Autodesk Inventor part; units mm, degrees
(part 2 of 3)
  spline S276 degree 2 poles (76.7813, 10.5842) (76.5936, 10.7868) (76.3861, 11.3302) (76.3861, 11.6859) knots 0 0 0 1 2 2 2
  spline S277 degree 2 poles (76.3861, 11.6859) (76.3861, 12.4269) (77.542, 13.4297) (78.4362, 13.4297) knots 0 0 0 1 2 2 2
  spline S278 degree 2 poles (78.4362, 13.4297) (78.95, 13.4297) (79.8589, 13.2272) (80.2492, 13.0345) knots 0 0 0 1 2 2 2
  line L270 (80.2492, 13.0345) -> (80.2492, 12.0662)
  line L271 (80.2492, 12.0662) -> (80.1899, 12.0662)
  spline S279 degree 2 poles (80.1899, 12.0662) (79.8984, 12.333) (78.9895, 12.7282) (78.4905, 12.7282) knots 0 0 0 1 2 2 2
  spline S280 degree 2 poles (78.4905, 12.7282) (77.9274, 12.7282) (77.2308, 12.1996) (77.2308, 11.7698) knots 0 0 0 1 2 2 2
  spline S281 degree 2 poles (77.2308, 11.7698) (77.2308, 11.3845) (77.6408, 10.9251) (78.0262, 10.8214) knots 0 0 0 1 2 2 2
  spline S282 degree 2 poles (78.0262, 10.8214) (78.283, 10.7522) (79.029, 10.5744) (79.276, 10.5003) knots 0 0 0 1 2 2 2
  spline S283 degree 2 poles (79.276, 10.5003) (79.9034, 10.3076) (80.4863, 9.532) (80.4863, 8.9639) knots 0 0 0 1 2 2 2
  spline S284 degree 2 poles (80.4863, 8.9639) (80.4863, 8.6033) (80.1948, 7.9117) (79.933, 7.6696) knots 0 0 0 1 2 2 2
  spline S285 degree 2 poles (79.933, 7.6696) (79.6416, 7.4029) (78.9006, 7.1163) (78.3423, 7.1163) knots 0 0 0 1 2 2 2
  line L272 (87.2097, 7.225) -> (84.2358, 7.225)
  line L273 (84.2358, 7.225) -> (84.2358, 7.8475)
  line L274 (84.2358, 7.8475) -> (85.3424, 7.8475)
  line L275 (85.3424, 7.8475) -> (85.3424, 11.9329)
  line L276 (85.3424, 11.9329) -> (84.2358, 11.9329)
  line L277 (84.2358, 11.9329) -> (84.2358, 12.4911)
  spline S286 degree 2 poles (84.2358, 12.4911) (84.8632, 12.4911) (85.456, 12.8468) (85.4955, 13.3408) knots 0 0 0 1 2 2 2
  line L278 (85.4955, 13.3408) -> (86.1278, 13.3408)
  line L279 (86.1278, 13.3408) -> (86.1278, 7.8475)
  line L280 (86.1278, 7.8475) -> (87.2097, 7.8475)
  line L281 (87.2097, 7.8475) -> (87.2097, 7.225)
  line L282 (87.8469, 7.225) -> (89.902, 13.321)
  line L283 (89.902, 13.321) -> (90.8999, 13.321)
  line L284 (90.8999, 13.321) -> (92.9549, 7.225)
  line L285 (92.9549, 7.225) -> (92.1003, 7.225)
  line L286 (92.1003, 7.225) -> (91.547, 8.9293)
  line L287 (91.547, 8.9293) -> (89.2203, 8.9293)
  line L288 (89.2203, 8.9293) -> (88.667, 7.225)
  line L289 (88.667, 7.225) -> (87.8469, 7.225)
  line L290 (91.3247, 9.6209) -> (90.3812, 12.4911)
  line L291 (90.3812, 12.4911) -> (89.4426, 9.6209)
  line L292 (89.4426, 9.6209) -> (91.3247, 9.6209)
  spline S287 degree 2 poles (97.8505, 7.1163) (97.1886, 7.1163) (96.2598, 7.393) (95.8498, 7.5906) knots 0 0 0 1 2 2 2
  line L293 (95.8498, 7.5906) -> (95.8498, 8.6082)
  line L294 (95.8498, 8.6082) -> (95.9091, 8.6082)
  spline S288 degree 2 poles (95.9091, 8.6082) (96.3092, 8.2328) (97.3219, 7.8178) (97.7912, 7.8178) knots 0 0 0 1 2 2 2
  spline S289 degree 2 poles (97.7912, 7.8178) (98.4631, 7.8178) (99.1497, 8.376) (99.1497, 8.8355) knots 0 0 0 1 2 2 2
  spline S290 degree 2 poles (99.1497, 8.8355) (99.1497, 9.201) (98.7891, 9.6555) (98.3989, 9.7691) knots 0 0 0 1 2 2 2
  spline S291 degree 2 poles (98.3989, 9.7691) (98.1173, 9.8482) (97.648, 9.9569) (97.2972, 10.0458) knots 0 0 0 1 2 2 2
  spline S292 degree 2 poles (97.2972, 10.0458) (96.9811, 10.1298) (96.4821, 10.3817) (96.2895, 10.5842) knots 0 0 0 1 2 2 2
  spline S293 degree 2 poles (96.2895, 10.5842) (96.1017, 10.7868) (95.8943, 11.3302) (95.8943, 11.6859) knots 0 0 0 1 2 2 2
  spline S294 degree 2 poles (95.8943, 11.6859) (95.8943, 12.4269) (97.0502, 13.4297) (97.9444, 13.4297) knots 0 0 0 1 2 2 2
  spline S295 degree 2 poles (97.9444, 13.4297) (98.4581, 13.4297) (99.3671, 13.2272) (99.7574, 13.0345) knots 0 0 0 1 2 2 2
  line L295 (99.7574, 13.0345) -> (99.7574, 12.0662)
  line L296 (99.7574, 12.0662) -> (99.6981, 12.0662)
  spline S296 degree 2 poles (99.6981, 12.0662) (99.4066, 12.333) (98.4977, 12.7282) (97.9987, 12.7282) knots 0 0 0 1 2 2 2
  spline S297 degree 2 poles (97.9987, 12.7282) (97.4356, 12.7282) (96.739, 12.1996) (96.739, 11.7698) knots 0 0 0 1 2 2 2
  spline S298 degree 2 poles (96.739, 11.7698) (96.739, 11.3845) (97.149, 10.9251) (97.5344, 10.8214) knots 0 0 0 1 2 2 2
  spline S299 degree 2 poles (97.5344, 10.8214) (97.7912, 10.7522) (98.5372, 10.5744) (98.7842, 10.5003) knots 0 0 0 1 2 2 2
  spline S300 degree 2 poles (98.7842, 10.5003) (99.4116, 10.3076) (99.9945, 9.532) (99.9945, 8.9639) knots 0 0 0 1 2 2 2
  spline S301 degree 2 poles (99.9945, 8.9639) (99.9945, 8.6033) (99.703, 7.9117) (99.4412, 7.6696) knots 0 0 0 1 2 2 2
  spline S302 degree 2 poles (99.4412, 7.6696) (99.1497, 7.4029) (98.4087, 7.1163) (97.8505, 7.1163) knots 0 0 0 1 2 2 2
  spline S303 degree 2 poles (102.7461, 7.1213) (101.6494, 7.1213) (100.444, 8.3513) (100.444, 9.4875) knots 0 0 0 1 2 2 2
  spline S304 degree 2 poles (100.444, 9.4875) (100.444, 10.604) (101.6148, 11.9279) (102.5584, 11.9279) knots 0 0 0 1 2 2 2
  spline S305 degree 2 poles (102.5584, 11.9279) (102.9832, 11.9279) (103.6402, 11.6809) (103.8823, 11.4191) knots 0 0 0 1 2 2 2
  spline S306 degree 2 poles (103.8823, 11.4191) (104.1293, 11.1573) (104.3911, 10.4015) (104.3911, 9.8531) knots 0 0 0 1 2 2 2
  line L297 (104.3911, 9.8531) -> (104.3911, 9.4332)
  line L298 (104.3911, 9.4332) -> (101.2246, 9.4332)
  spline S307 degree 2 poles (101.2246, 9.4332) (101.2246, 8.6379) (102.0248, 7.7931) (102.7362, 7.7931) knots 0 0 0 1 2 2 2
  spline S308 degree 2 poles (102.7362, 7.7931) (102.9881, 7.7931) (103.4772, 7.9067) (103.6748, 7.9957) knots 0 0 0 1 2 2 2
  spline S309 degree 2 poles (103.6748, 7.9957) (103.8823, 8.0945) (104.1688, 8.2674) (104.2627, 8.3464) knots 0 0 0 1 2 2 2
  line L299 (104.2627, 8.3464) -> (104.3071, 8.3464)
  line L300 (104.3071, 8.3464) -> (104.3071, 7.5066)
  spline S310 degree 2 poles (104.3071, 7.5066) (104.1738, 7.4523) (103.7687, 7.2942) (103.6106, 7.2497) knots 0 0 0 1 2 2 2
  spline S311 degree 2 poles (103.6106, 7.2497) (103.3883, 7.1855) (103.0227, 7.1213) (102.7461, 7.1213) knots 0 0 0 1 2 2 2
  spline S312 degree 2 poles (103.6402, 10.0211) (103.6304, 10.3323) (103.5019, 10.7868) (103.3784, 10.9399) knots 0 0 0 1 2 2 2
  spline S313 degree 2 poles (103.3784, 10.9399) (103.245, 11.1128) (102.8251, 11.2956) (102.5139, 11.2956) knots 0 0 0 1 2 2 2
  spline S314 degree 2 poles (102.5139, 11.2956) (102.2076, 11.2956) (101.7778, 11.1128) (101.6, 10.935) knots 0 0 0 1 2 2 2
  spline S315 degree 2 poles (101.6, 10.935) (101.4271, 10.7522) (101.2493, 10.3125) (101.2246, 10.0211) knots 0 0 0 1 2 2 2
  line L301 (101.2246, 10.0211) -> (103.6402, 10.0211)
  spline S316 degree 2 poles (106.9896, 7.1213) (106.5153, 7.1213) (105.7299, 7.4127) (105.4483, 7.7091) knots 0 0 0 1 2 2 2
  spline S317 degree 2 poles (105.4483, 7.7091) (105.1667, 8.0006) (104.8555, 8.8997) (104.8555, 9.5024) knots 0 0 0 1 2 2 2
  spline S318 degree 2 poles (104.8555, 9.5024) (104.8555, 10.1051) (105.1766, 10.9844) (105.4483, 11.2808) knots 0 0 0 1 2 2 2
  spline S319 degree 2 poles (105.4483, 11.2808) (105.72, 11.5821) (106.5252, 11.9032) (106.9896, 11.9032) knots 0 0 0 1 2 2 2
  spline S320 degree 2 poles (106.9896, 11.9032) (107.365, 11.9032) (108.0665, 11.6908) (108.3382, 11.5525) knots 0 0 0 1 2 2 2
  line L302 (108.3382, 11.5525) -> (108.3382, 10.688)
  line L303 (108.3382, 10.688) -> (108.2937, 10.688)
  spline S321 degree 2 poles (108.2937, 10.688) (108.2098, 10.7571) (107.9529, 10.935) (107.7701, 11.0288) knots 0 0 0 1 2 2 2
  spline S322 degree 2 poles (107.7701, 11.0288) (107.6071, 11.1079) (107.1724, 11.2314) (106.9748, 11.2314) knots 0 0 0 1 2 2 2
  spline S323 degree 2 poles (106.9748, 11.2314) (106.377, 11.2314) (105.6508, 10.3274) (105.6508, 9.5024) knots 0 0 0 1 2 2 2
  spline S324 degree 2 poles (105.6508, 9.5024) (105.6508, 8.6971) (106.3523, 7.7931) (106.9748, 7.7931) knots 0 0 0 1 2 2 2
  spline S325 degree 2 poles (106.9748, 7.7931) (107.3502, 7.7931) (108.0319, 8.1043) (108.2937, 8.3464) knots 0 0 0 1 2 2 2
  line L304 (108.2937, 8.3464) -> (108.3382, 8.3464)
  line L305 (108.3382, 8.3464) -> (108.3382, 7.4819)
  spline S326 degree 2 poles (108.3382, 7.4819) (108.2246, 7.4276) (107.8788, 7.2744) (107.7405, 7.2398) knots 0 0 0 1 2 2 2
  spline S327 degree 2 poles (107.7405, 7.2398) (107.5429, 7.1806) (107.2316, 7.1213) (106.9896, 7.1213) knots 0 0 0 1 2 2 2
  spline S328 degree 2 poles (110.4229, 7.1361) (109.7955, 7.1361) (109.0891, 7.8524) (109.0891, 8.628) knots 0 0 0 1 2 2 2
  line L306 (109.0891, 8.628) -> (109.0891, 11.1622)
  line L307 (109.0891, 11.1622) -> (108.5704, 11.1622)
  line L308 (108.5704, 11.1622) -> (108.5704, 11.7995)
  line L309 (108.5704, 11.7995) -> (109.0891, 11.7995)
  line L310 (109.0891, 11.7995) -> (109.0891, 13.1135)
  line L311 (109.0891, 13.1135) -> (109.8597, 13.1135)
  line L312 (109.8597, 13.1135) -> (109.8597, 11.7995)
  line L313 (109.8597, 11.7995) -> (111.2775, 11.7995)
  line L314 (111.2775, 11.7995) -> (111.2775, 11.1622)
  line L315 (111.2775, 11.1622) -> (109.8597, 11.1622)
  line L316 (109.8597, 11.1622) -> (109.8597, 8.9837)
  spline S329 degree 2 poles (109.8597, 8.9837) (109.8597, 8.6379) (109.8844, 8.2575) (109.9684, 8.0945) knots 0 0 0 1 2 2 2
  spline S330 degree 2 poles (109.9684, 8.0945) (110.0376, 7.9512) (110.3488, 7.8079) (110.6156, 7.8079) knots 0 0 0 1 2 2 2
  spline S331 degree 2 poles (110.6156, 7.8079) (110.8033, 7.8079) (111.154, 7.9216) (111.2331, 7.9561) knots 0 0 0 1 2 2 2
  line L317 (111.2331, 7.9561) -> (111.2775, 7.9561)
  line L318 (111.2775, 7.9561) -> (111.2775, 7.2645)
  spline S332 degree 2 poles (111.2775, 7.2645) (111.0602, 7.2053) (110.6156, 7.1361) (110.4229, 7.1361) knots 0 0 0 1 2 2 2
  line L319 (112.6311, 7.225) -> (111.8604, 7.225)
  line L320 (111.8604, 7.225) -> (111.8604, 11.7995)
  line L321 (111.8604, 11.7995) -> (112.6311, 11.7995)
  line L322 (112.6311, 11.7995) -> (112.6311, 7.225)
  line L323 (112.6854, 12.5602) -> (111.811, 12.5602)
  line L324 (111.811, 12.5602) -> (111.811, 13.3605)
  line L325 (111.811, 13.3605) -> (112.6854, 13.3605)
  line L326 (112.6854, 13.3605) -> (112.6854, 12.5602)
  spline S333 degree 2 poles (117.5217, 9.5122) (117.5217, 8.3563) (116.4102, 7.0966) (115.4815, 7.0966) knots 0 0 0 1 2 2 2
  spline S334 degree 2 poles (115.4815, 7.0966) (114.5281, 7.0966) (113.4363, 8.3958) (113.4363, 9.5122) knots 0 0 0 1 2 2 2
  spline S335 degree 2 poles (113.4363, 9.5122) (113.4363, 10.6583) (114.5626, 11.9279) (115.4815, 11.9279) knots 0 0 0 1 2 2 2
  spline S336 degree 2 poles (115.4815, 11.9279) (116.4102, 11.9279) (117.5217, 10.6633) (117.5217, 9.5122) knots 0 0 0 1 2 2 2
  spline S337 degree 2 poles (116.7264, 9.5122) (116.7264, 10.4015) (116.0792, 11.266) (115.4815, 11.266) knots 0 0 0 1 2 2 2
  spline S338 degree 2 poles (115.4815, 11.266) (114.8837, 11.266) (114.2317, 10.4015) (114.2317, 9.5122) knots 0 0 0 1 2 2 2
  spline S339 degree 2 poles (114.2317, 9.5122) (114.2317, 8.6477) (114.8837, 7.7585) (115.4815, 7.7585) knots 0 0 0 1 2 2 2
  spline S340 degree 2 poles (115.4815, 7.7585) (116.0743, 7.7585) (116.7264, 8.6329) (116.7264, 9.5122) knots 0 0 0 1 2 2 2
  line L327 (121.9035, 7.225) -> (121.1329, 7.225)
  line L328 (121.1329, 7.225) -> (121.1329, 9.8334)
  spline S341 degree 2 poles (121.1329, 9.8334) (121.1329, 10.1495) (121.0736, 10.6929) (120.9847, 10.8559) knots 0 0 0 1 2 2 2
  spline S342 degree 2 poles (120.9847, 10.8559) (120.8908, 11.0288) (120.5549, 11.1968) (120.2684, 11.1968) knots 0 0 0 1 2 2 2
  spline S343 degree 2 poles (120.2684, 11.1968) (119.9819, 11.1968) (119.3742, 10.8905) (119.0828, 10.6435) knots 0 0 0 1 2 2 2
  line L329 (119.0828, 10.6435) -> (119.0828, 7.225)
  line L330 (119.0828, 7.225) -> (118.3121, 7.225)
  line L331 (118.3121, 7.225) -> (118.3121, 11.7995)
  line L332 (118.3121, 11.7995) -> (119.0828, 11.7995)
  line L333 (119.0828, 11.7995) -> (119.0828, 11.2907)
  spline S344 degree 2 poles (119.0828, 11.2907) (119.4286, 11.6019) (120.0955, 11.9279) (120.4709, 11.9279) knots 0 0 0 1 2 2 2
  spline S345 degree 2 poles (120.4709, 11.9279) (121.1428, 11.9279) (121.9035, 11.0387) (121.9035, 10.194) knots 0 0 0 1 2 2 2
  line L334 (121.9035, 10.194) -> (121.9035, 7.225)
  spline S346 degree 2 poles (129.7977, 9.0973) (129.7977, 8.6428) (129.4519, 7.9463) (129.1654, 7.719) knots 0 0 0 1 2 2 2
  spline S347 degree 2 poles (129.1654, 7.719) (128.8196, 7.4523) (128.0341, 7.225) (127.4117, 7.225) knots 0 0 0 1 2 2 2
  line L335 (127.4117, 7.225) -> (125.6629, 7.225)
  line L336 (125.6629, 7.225) -> (125.6629, 13.321)
  line L337 (125.6629, 13.321) -> (127.2783, 13.321)
  spline S348 degree 2 poles (127.2783, 13.321) (127.9304, 13.321) (128.5825, 13.237) (128.8789, 13.074) knots 0 0 0 1 2 2 2
  spline S349 degree 2 poles (128.8789, 13.074) (129.2098, 12.9011) (129.5112, 12.333) (129.5112, 11.9477) knots 0 0 0 1 2 2 2
  spline S350 degree 2 poles (129.5112, 11.9477) (129.5112, 11.5179) (129.0567, 10.8362) (128.6566, 10.6435) knots 0 0 0 1 2 2 2
  line L338 (128.6566, 10.6435) -> (128.6566, 10.6139)
  spline S351 degree 2 poles (128.6566, 10.6139) (129.2, 10.4657) (129.7977, 9.6802) (129.7977, 9.0973) knots 0 0 0 1 2 2 2
  spline S352 degree 2 poles (128.953, 9.0627) (128.953, 9.4085) (128.7554, 9.8531) (128.459, 10.0112) knots 0 0 0 1 2 2 2
  spline S353 degree 2 poles (128.459, 10.0112) (128.2663, 10.11) (127.8118, 10.1693) (127.3919, 10.1693) knots 0 0 0 1 2 2 2
  line L339 (127.3919, 10.1693) -> (126.4731, 10.1693)
  line L340 (126.4731, 10.1693) -> (126.4731, 7.9166)
  line L341 (126.4731, 7.9166) -> (127.1301, 7.9166)
  spline S354 degree 2 poles (127.1301, 7.9166) (127.6636, 7.9166) (128.2762, 8.0154) (128.5133, 8.1735) knots 0 0 0 1 2 2 2
  spline S355 degree 2 poles (128.5133, 8.1735) (128.7405, 8.3365) (128.953, 8.7416) (128.953, 9.0627) knots 0 0 0 1 2 2 2
  spline S356 degree 2 poles (128.6664, 11.8341) (128.6664, 12.0514) (128.5182, 12.3775) (128.3552, 12.4713) knots 0 0 0 1 2 2 2
  spline S357 degree 2 poles (128.3552, 12.4713) (128.1576, 12.58) (127.6784, 12.6294) (127.2486, 12.6294) knots 0 0 0 1 2 2 2
  line L342 (127.2486, 12.6294) -> (126.4731, 12.6294)
  line L343 (126.4731, 12.6294) -> (126.4731, 10.8461)
  line L344 (126.4731, 10.8461) -> (127.3919, 10.8461)
  spline S358 degree 2 poles (127.3919, 10.8461) (127.7723, 10.8461) (128.1329, 10.9251) (128.3256, 11.0486) knots 0 0 0 1 2 2 2
  spline S359 degree 2 poles (128.3256, 11.0486) (128.5133, 11.1672) (128.6664, 11.5475) (128.6664, 11.8341) knots 0 0 0 1 2 2 2
  spline S360 degree 2 poles (134.224, 10.273) (134.224, 8.6329) (133.2705, 7.0966) (132.2776, 7.0966) knots 0 0 0 1 2 2 2
  spline S361 degree 2 poles (132.2776, 7.0966) (131.2698, 7.0966) (130.3263, 8.6626) (130.3263, 10.2681) knots 0 0 0 1 2 2 2
  spline S362 degree 2 poles (130.3263, 10.2681) (130.3263, 11.918) (131.2797, 13.4445) (132.2776, 13.4445) knots 0 0 0 1 2 2 2
  spline S363 degree 2 poles (132.2776, 13.4445) (133.2804, 13.4445) (134.224, 11.8637) (134.224, 10.273) knots 0 0 0 1 2 2 2
  spline S364 degree 2 poles (133.1767, 8.4156) (133.2952, 8.7169) (133.394, 9.6456) (133.394, 10.273) knots 0 0 0 1 2 2 2
  spline S365 degree 2 poles (133.394, 10.273) (133.394, 10.9004) (133.2952, 11.8242) (133.1717, 12.1354) knots 0 0 0 1 2 2 2
  spline S366 degree 2 poles (133.1717, 12.1354) (133.0482, 12.4466) (132.6185, 12.7677) (132.2776, 12.7677) knots 0 0 0 1 2 2 2
  spline S367 degree 2 poles (132.2776, 12.7677) (131.9367, 12.7677) (131.4971, 12.4466) (131.3686, 12.1255) knots 0 0 0 1 2 2 2
  spline S368 degree 2 poles (131.3686, 12.1255) (131.2451, 11.8143) (131.1562, 10.8658) (131.1562, 10.2681) knots 0 0 0 1 2 2 2
  spline S369 degree 2 poles (131.1562, 10.2681) (131.1562, 9.6259) (131.2353, 8.7663) (131.3637, 8.4304) knots 0 0 0 1 2 2 2
  spline S370 degree 2 poles (131.3637, 8.4304) (131.4823, 8.1142) (131.9219, 7.7734) (132.2776, 7.7734) knots 0 0 0 1 2 2 2
  spline S371 degree 2 poles (132.2776, 7.7734) (132.6135, 7.7734) (133.0532, 8.0945) (133.1767, 8.4156) knots 0 0 0 1 2 2 2
  spline S372 degree 2 poles (136.6495, 12.743) (136.4272, 12.743) (135.9876, 12.6343) (135.7751, 12.5504) knots 0 0 0 1 2 2 2
  spline S373 degree 2 poles (135.7751, 12.5504) (135.5775, 12.4664) (135.2861, 12.2885) (135.1725, 12.2095) knots 0 0 0 1 2 2 2
  line L345 (135.1725, 12.2095) -> (135.1231, 12.2095)
  line L346 (135.1231, 12.2095) -> (135.1231, 13.074)
  spline S374 degree 2 poles (135.1231, 13.074) (135.3898, 13.2173) (136.3037, 13.4495) (136.7138, 13.4495) knots 0 0 0 1 2 2 2
  spline S375 degree 2 poles (136.7138, 13.4495) (137.1287, 13.4495) (137.7462, 13.2815) (137.9982, 13.1037) knots 0 0 0 1 2 2 2
  spline S376 degree 2 poles (137.9982, 13.1037) (138.2649, 12.911) (138.5416, 12.3528) (138.5416, 11.9773) knots 0 0 0 1 2 2 2
  spline S377 degree 2 poles (138.5416, 11.9773) (138.5416, 11.4734) (137.8796, 10.7127) (137.4152, 10.6139) knots 0 0 0 1 2 2 2
  line L347 (137.4152, 10.6139) -> (137.4152, 10.5546)
  spline S378 degree 2 poles (137.4152, 10.5546) (137.6079, 10.5151) (138.0476, 10.3372) (138.2353, 10.1594) knots 0 0 0 1 2 2 2
  spline S379 degree 2 poles (138.2353, 10.1594) (138.423, 9.9865) (138.6601, 9.4332) (138.6601, 9.0331) knots 0 0 0 1 2 2 2
  spline S380 degree 2 poles (138.6601, 9.0331) (138.6601, 8.623) (138.3785, 7.9265) (138.1217, 7.6597) knots 0 0 0 1 2 2 2
  spline S381 degree 2 poles (138.1217, 7.6597) (137.8549, 7.3831) (137.0991, 7.0966) (136.6199, 7.0966) knots 0 0 0 1 2 2 2
  spline S382 degree 2 poles (136.6199, 7.0966) (136.1605, 7.0966) (135.2614, 7.3189) (134.9551, 7.472) knots 0 0 0 1 2 2 2
  line L348 (134.9551, 7.472) -> (134.9551, 8.3365)
  line L349 (134.9551, 8.3365) -> (135.0144, 8.3365)
  spline S383 degree 2 poles (135.0144, 8.3365) (135.2713, 8.1488) (136.1407, 7.803) (136.5705, 7.803) knots 0 0 0 1 2 2 2
  spline S384 degree 2 poles (136.5705, 7.803) (136.8224, 7.803) (137.3263, 7.9611) (137.4943, 8.1439) knots 0 0 0 1 2 2 2
  spline S385 degree 2 poles (137.4943, 8.1439) (137.6573, 8.3266) (137.8302, 8.7614) (137.8302, 9.0923) knots 0 0 0 1 2 2 2
  spline S386 degree 2 poles (137.8302, 9.0923) (137.8302, 9.4233) (137.6375, 9.8531) (137.4646, 9.9766) knots 0 0 0 1 2 2 2
  spline S387 degree 2 poles (137.4646, 9.9766) (137.2917, 10.1001) (136.8224, 10.194) (136.5458, 10.194) knots 0 0 0 1 2 2 2
  line L350 (136.5458, 10.194) -> (136.2, 10.194)
  line L351 (136.2, 10.194) -> (136.2, 10.8708)
  line L352 (136.2, 10.8708) -> (136.4717, 10.8708)
  spline S388 degree 2 poles (136.4717, 10.8708) (137.02, 10.8708) (137.7116, 11.3944) (137.7116, 11.8933) knots 0 0 0 1 2 2 2
  spline S389 degree 2 poles (137.7116, 11.8933) (137.7116, 12.1255) (137.5338, 12.4565) (137.3905, 12.5553) knots 0 0 0 1 2 2 2
  spline S390 degree 2 poles (137.3905, 12.5553) (137.2374, 12.659) (136.862, 12.743) (136.6495, 12.743) knots 0 0 0 1 2 2 2
  dimension "d2" = 50.8
  dimension "d3" = 203.2
  dimension "d4" = 50.8
  dimension "d5" = 101.6
  dimension "d6" = 8.128
  dimension "d7" = 21.336
  constraints: 2 other
  measures "d2" distance between parallel lines of L2 L7
  measures "d3" distance of L2.end L0.start
  measures "d4" distance of L1.end L2.end
  measures "d5" distance of L5.end L6.end
  measures "d6" distance of L6.end L4.start
  measures "d7" distance between parallel lines of L1 L4
extrude "Extrusion2" cut sketch "Sketch2" against normal blind 5.08 contours S0 S1 L8 L9 S2 S3 S4 L10 L11 L12 L13 L14 | L15 L16 S5 S6 S7 L17 L18 L19 S8 S9 S10 L20 L21 L22 | S11 L23 L24 S12 S13 S14 S15 S16 S17 S18 S19 S20 L25 L26 S21 S22 S23 S24 S25 S26 S27 | S28 L27 L28 L29 L30 L31 L32 L33 L34 L35 L36 L37 S29 S30 S31 L38 L39 S32 | L40 L41 L42 L43 | L44 L45 L46 L47 | L48 L49 S33 S34 S35 L50 L51 L52 L53 L54 S36 S37 L55 | L56 L57 L58 L59 L60 L61 L62 L63 | L67 L68 L69 L70 | L71 L72 L73 L74 | S38 S39 S40 S41 L75 L76 S42 S43 S44 L77 L78 S45 S46 | L80 L81 S51 S52 S53 L82 L83 L84 L85 L86 S54 S55 L87 | L88 L89 L90 L91 L92 L93 L94 L95 | L99 L100 L101 L102 L103 L104 S56 L105 L106 L107 L108 | L109 L110 L111 L112 L113 L114 L115 L116 L117 L118 L119 | S57 S58 S59 L123 L124 S60 S61 S62 S63 S64 S65 S66 L125 L126 L127 L128 L129 S67 S68 S69 | S70 S71 S72 S73 S74 S75 S76 L130 L131 S77 S78 S79 S80 S81 | S89 S90 S91 S92 S93 S94 S95 L132 L133 S96 S97 S98 S99 S100 | S108 S109 S110 S111 | L134 L135 L136 L137 L138 L139 L140 | L141 L142 L143 L144 L145 L146 S120 L147 L148 L149 L150 | S121 S122 L151 L152 S123 S124 S125 L153 L154 L155 L156 L157 | L158 L159 L160 L161 | S126 S127 L162 L163 L164 L165 L166 S128 S129 | S134 S135 S136 S137 S138 S139 L168 S140 S141 S142 L169 L170 S143 S144 S145 L171 L172 L173 | L175 L176 L177 L178 | L179 L180 L181 L182 | S150 S151 S152 S153 L183 L184 S154 S155 S156 L185 L186 S157 S158 | L188 L189 S163 S164 S165 L190 L191 L192 L193 L194 S166 S167 L195 | S168 L196 L197 S169 S170 S171 S172 L198 L199 L200 L201 S173 S174 S175 S176 S177 L202 S178 S179 S180 S181 | L204 L205 S186 S187 S188 L206 L207 L208 S189 S190 S191 L209 L210 L211 | S192 S193 S194 S195 S196 L212 L213 S197 S198 S199 S200 S201 L214 L215 S202 S203 | S204 L216 L217 S205 S206 S207 S208 S209 S210 S211 S212 S213 L218 L219 S214 S215 S216 S217 S218 S219 S220 | L220 L221 S221 S222 S223 S224 S225 S226 S227 L222 L223 L224 | L226 L227 L228 L229 | S232 S233 S234 S235 L230 L231 S236 S237 S238 L232 L233 S239 S240 | L235 L236 S245 S246 S247 S248 S249 S250 S251 L237 L238 L239 | L241 L242 S256 S257 S258 L243 L244 L245 S259 S260 S261 L246 L247 L248 | L249 L250 L251 L252 L253 L254 L255 L256 L257 L258 L259 L260 L261 | S262 S263 L262 L263 L264 S264 S265 S266 S267 L265 L266 L267 S268 S269 | S270 L268 L269 S271 S272 S273 S274 S275 S276 S277 S278 L270 L271 S279 S280 S281 S282 S283 S284 S285 | L272 L273 L274 L275 L276 L277 S286 L278 L279 L280 L281 | L282 L283 L284 L285 L286 L287 L288 L289 | S287 L293 L294 S288 S289 S290 S291 S292 S293 S294 S295 L295 L296 S296 S297 S298 S299 S300 S301 S302 | S303 S304 S305 S306 L297 L298 S307 S308 S309 L299 L300 S310 S311 | S316 S317 S318 S319 S320 L302 L303 S321 S322 S323 S324 S325 L304 L305 S326 S327 | S328 L306 L307 L308 L309 L310 L311 L312 L313 L314 L315 L316 S329 S330 S331 L317 L318 S332 | L319 L320 L321 L322 | L323 L324 L325 L326 | S333 S334 S335 S336 | L327 L328 S341 S342 S343 L329 L330 L331 L332 L333 S344 S345 L334 | S346 S347 L335 L336 L337 S348 S349 S350 L338 S351 | S360 S361 S362 S363 | S372 S373 L345 L346 S374 S375 S376 S377 L347 S378 S379 S380 S381 S382 L348 L349 S383 S384 S385 S386 S387 L350 L351 L352 S388 S389 S390
sketch "Sketch3" plane through (0, 0, 50.8) normal (0, 0, 1) x (1, 0, 0)
  line L0 (0, 0) -> (203.2, 0) projected
  line L1 (0, 0) -> (0, -25.4) projected
  line L2 (203.2, -25.4) -> (0, -25.4) projected
  line L3 (203.2, 0) -> (203.2, -25.4) projected
  line L4 (50.8, -8.636) -> (152.4, -8.636) construction
  line L5 (152.4, -8.636) -> (152.4, -16.764) construction
  line L6 (152.4, -16.764) -> (50.8, -16.764) construction
  line L7 (50.8, -16.764) -> (50.8, -8.636) construction
  line L8 (77.3469, -15.748) -> (73.8148, -15.748)
  line L9 (73.8148, -15.748) -> (73.8148, -9.652)
  line L10 (73.8148, -9.652) -> (74.625, -9.652)
  line L11 (74.625, -9.652) -> (74.625, -15.0268)
  line L12 (74.625, -15.0268) -> (77.3469, -15.0268)
  line L13 (77.3469, -15.0268) -> (77.3469, -15.748)
  line L14 (80.1084, -15.748) -> (77.7471, -15.748)
  line L15 (77.7471, -15.748) -> (77.7471, -15.1256)
  line L16 (77.7471, -15.1256) -> (78.5226, -15.1256)
  line L17 (78.5226, -15.1256) -> (78.5226, -10.2744)
  line L18 (78.5226, -10.2744) -> (77.7471, -10.2744)
  line L19 (77.7471, -10.2744) -> (77.7471, -9.652)
  line L20 (77.7471, -9.652) -> (80.1084, -9.652)
  line L21 (80.1084, -9.652) -> (80.1084, -10.2744)
  line L22 (80.1084, -10.2744) -> (79.3328, -10.2744)
  line L23 (79.3328, -10.2744) -> (79.3328, -15.1256)
  line L24 (79.3328, -15.1256) -> (80.1084, -15.1256)
  line L25 (80.1084, -15.1256) -> (80.1084, -15.748)
  spline S0 degree 2 poles (85.246, -13.8757) (85.246, -14.3302) (84.9002, -15.0268) (84.6137, -15.254) knots 0 0 0 1 2 2 2
  spline S1 degree 2 poles (84.6137, -15.254) (84.2679, -15.5208) (83.4824, -15.748) (82.86, -15.748) knots 0 0 0 1 2 2 2
  line L26 (82.86, -15.748) -> (81.1112, -15.748)
  line L27 (81.1112, -15.748) -> (81.1112, -9.652)
  line L28 (81.1112, -9.652) -> (82.7266, -9.652)
  spline S2 degree 2 poles (82.7266, -9.652) (83.3787, -9.652) (84.0308, -9.736) (84.3272, -9.899) knots 0 0 0 1 2 2 2
  spline S3 degree 2 poles (84.3272, -9.899) (84.6582, -10.0719) (84.9595, -10.64) (84.9595, -11.0253) knots 0 0 0 1 2 2 2
  spline S4 degree 2 poles (84.9595, -11.0253) (84.9595, -11.4551) (84.505, -12.1368) (84.1049, -12.3295) knots 0 0 0 1 2 2 2
  line L29 (84.1049, -12.3295) -> (84.1049, -12.3591)
  spline S5 degree 2 poles (84.1049, -12.3591) (84.6483, -12.5073) (85.246, -13.2928) (85.246, -13.8757) knots 0 0 0 1 2 2 2
  spline S6 degree 2 poles (84.4013, -13.9103) (84.4013, -13.5645) (84.2037, -13.1199) (83.9073, -12.9618) knots 0 0 0 1 2 2 2
  spline S7 degree 2 poles (83.9073, -12.9618) (83.7146, -12.863) (83.2601, -12.8037) (82.8402, -12.8037) knots 0 0 0 1 2 2 2
  line L30 (82.8402, -12.8037) -> (81.9214, -12.8037)
  line L31 (81.9214, -12.8037) -> (81.9214, -15.0564)
  line L32 (81.9214, -15.0564) -> (82.5784, -15.0564)
  spline S8 degree 2 poles (82.5784, -15.0564) (83.1119, -15.0564) (83.7245, -14.9576) (83.9616, -14.7995) knots 0 0 0 1 2 2 2
  spline S9 degree 2 poles (83.9616, -14.7995) (84.1889, -14.6365) (84.4013, -14.2314) (84.4013, -13.9103) knots 0 0 0 1 2 2 2
  spline S10 degree 2 poles (84.1148, -11.1389) (84.1148, -10.9216) (83.9666, -10.5955) (83.8035, -10.5017) knots 0 0 0 1 2 2 2
  spline S11 degree 2 poles (83.8035, -10.5017) (83.6059, -10.393) (83.1267, -10.3436) (82.697, -10.3436) knots 0 0 0 1 2 2 2
  line L33 (82.697, -10.3436) -> (81.9214, -10.3436)
  line L34 (81.9214, -10.3436) -> (81.9214, -12.127)
  line L35 (81.9214, -12.127) -> (82.8402, -12.127)
  spline S12 degree 2 poles (82.8402, -12.127) (83.2206, -12.127) (83.5812, -12.0479) (83.7739, -11.9244) knots 0 0 0 1 2 2 2
  spline S13 degree 2 poles (83.7739, -11.9244) (83.9616, -11.8059) (84.1148, -11.4255) (84.1148, -11.1389) knots 0 0 0 1 2 2 2
  line L36 (90.769, -15.748) -> (89.7167, -15.748)
  line L37 (89.7167, -15.748) -> (87.7901, -13.3224)
  line L38 (87.7901, -13.3224) -> (86.8614, -13.3224)
  line L39 (86.8614, -13.3224) -> (86.8614, -15.748)
  line L40 (86.8614, -15.748) -> (86.0512, -15.748)
  line L41 (86.0512, -15.748) -> (86.0512, -9.652)
  line L42 (86.0512, -9.652) -> (87.6222, -9.652)
  spline S14 degree 2 poles (87.6222, -9.652) (88.1458, -9.652) (88.8522, -9.7656) (89.1733, -9.9731) knots 0 0 0 1 2 2 2
  spline S15 degree 2 poles (89.1733, -9.9731) (89.4944, -10.1806) (89.865, -10.8277) (89.865, -11.3069) knots 0 0 0 1 2 2 2
  spline S16 degree 2 poles (89.865, -11.3069) (89.865, -11.9738) (89.1832, -12.8778) (88.6003, -13.0952) knots 0 0 0 1 2 2 2
  line L43 (88.6003, -13.0952) -> (90.769, -15.748)
  spline S17 degree 2 poles (89.0202, -11.3711) (89.0202, -11.1044) (88.8325, -10.6943) (88.6349, -10.561) knots 0 0 0 1 2 2 2
  spline S18 degree 2 poles (88.6349, -10.561) (88.462, -10.4473) (88.0026, -10.3535) (87.6666, -10.3535) knots 0 0 0 1 2 2 2
  line L44 (87.6666, -10.3535) -> (86.8614, -10.3535)
  line L45 (86.8614, -10.3535) -> (86.8614, -12.6457)
  line L46 (86.8614, -12.6457) -> (87.5728, -12.6457)
  spline S19 degree 2 poles (87.5728, -12.6457) (87.9235, -12.6457) (88.4817, -12.5222) (88.6744, -12.3295) knots 0 0 0 1 2 2 2
  spline S20 degree 2 poles (88.6744, -12.3295) (88.8522, -12.1615) (89.0202, -11.6873) (89.0202, -11.3711) knots 0 0 0 1 2 2 2
  line L47 (90.5961, -15.748) -> (92.6511, -9.652)
  line L48 (92.6511, -9.652) -> (93.649, -9.652)
  line L49 (93.649, -9.652) -> (95.7041, -15.748)
  line L50 (95.7041, -15.748) -> (94.8494, -15.748)
  line L51 (94.8494, -15.748) -> (94.2962, -14.0437)
  line L52 (94.2962, -14.0437) -> (91.9694, -14.0437)
  line L53 (91.9694, -14.0437) -> (91.4161, -15.748)
  line L54 (91.4161, -15.748) -> (90.5961, -15.748)
  line L55 (94.0739, -13.3521) -> (93.1303, -10.4819)
  line L56 (93.1303, -10.4819) -> (92.1917, -13.3521)
  line L57 (92.1917, -13.3521) -> (94.0739, -13.3521)
  line L58 (100.9998, -15.748) -> (99.9476, -15.748)
  line L59 (99.9476, -15.748) -> (98.0209, -13.3224)
  line L60 (98.0209, -13.3224) -> (97.0922, -13.3224)
  line L61 (97.0922, -13.3224) -> (97.0922, -15.748)
  line L62 (97.0922, -15.748) -> (96.2821, -15.748)
  line L63 (96.2821, -15.748) -> (96.2821, -9.652)
  line L64 (96.2821, -9.652) -> (97.853, -9.652)
  spline S21 degree 2 poles (97.853, -9.652) (98.3766, -9.652) (99.0831, -9.7656) (99.4042, -9.9731) knots 0 0 0 1 2 2 2
  spline S22 degree 2 poles (99.4042, -9.9731) (99.7253, -10.1806) (100.0958, -10.8277) (100.0958, -11.3069) knots 0 0 0 1 2 2 2
  spline S23 degree 2 poles (100.0958, -11.3069) (100.0958, -11.9738) (99.414, -12.8778) (98.8311, -13.0952) knots 0 0 0 1 2 2 2
  line L65 (98.8311, -13.0952) -> (100.9998, -15.748)
  spline S24 degree 2 poles (99.251, -11.3711) (99.251, -11.1044) (99.0633, -10.6943) (98.8657, -10.561) knots 0 0 0 1 2 2 2
  spline S25 degree 2 poles (98.8657, -10.561) (98.6928, -10.4473) (98.2334, -10.3535) (97.8974, -10.3535) knots 0 0 0 1 2 2 2
  line L66 (97.8974, -10.3535) -> (97.0922, -10.3535)
  line L67 (97.0922, -10.3535) -> (97.0922, -12.6457)
  line L68 (97.0922, -12.6457) -> (97.8036, -12.6457)
  spline S26 degree 2 poles (97.8036, -12.6457) (98.1543, -12.6457) (98.7125, -12.5222) (98.9052, -12.3295) knots 0 0 0 1 2 2 2
  spline S27 degree 2 poles (98.9052, -12.3295) (99.0831, -12.1615) (99.251, -11.6873) (99.251, -11.3711) knots 0 0 0 1 2 2 2
  line L69 (105.7521, -9.652) -> (103.6921, -13.0507)
  line L70 (103.6921, -13.0507) -> (103.6921, -15.748)
  line L71 (103.6921, -15.748) -> (102.8819, -15.748)
  line L72 (102.8819, -15.748) -> (102.8819, -13.1347)
  line L73 (102.8819, -13.1347) -> (100.8219, -9.652)
  line L74 (100.8219, -9.652) -> (101.721, -9.652)
  line L75 (101.721, -9.652) -> (103.292, -12.3344)
  line L76 (103.292, -12.3344) -> (104.8925, -9.652)
  line L77 (104.8925, -9.652) -> (105.7521, -9.652)
  line L78 (115.7655, -9.652) -> (114.2341, -15.748)
  line L79 (114.2341, -15.748) -> (113.3252, -15.748)
  line L80 (113.3252, -15.748) -> (112.0852, -10.6894)
  line L81 (112.0852, -10.6894) -> (110.8798, -15.748)
  line L82 (110.8798, -15.748) -> (109.9808, -15.748)
  line L83 (109.9808, -15.748) -> (108.4247, -9.652)
  line L84 (108.4247, -9.652) -> (109.2595, -9.652)
  line L85 (109.2595, -9.652) -> (110.4846, -14.7057)
  line L86 (110.4846, -14.7057) -> (111.6999, -9.652)
  line L87 (111.6999, -9.652) -> (112.5249, -9.652)
  line L88 (112.5249, -9.652) -> (113.75, -14.7649)
  line L89 (113.75, -14.7649) -> (114.9702, -9.652)
  line L90 (114.9702, -9.652) -> (115.7655, -9.652)
  line L91 (115.8347, -15.748) -> (117.8898, -9.652)
  line L92 (117.8898, -9.652) -> (118.8876, -9.652)
  line L93 (118.8876, -9.652) -> (120.9427, -15.748)
  line L94 (120.9427, -15.748) -> (120.0881, -15.748)
  line L95 (120.0881, -15.748) -> (119.5348, -14.0437)
  line L96 (119.5348, -14.0437) -> (117.208, -14.0437)
  line L97 (117.208, -14.0437) -> (116.6547, -15.748)
  line L98 (116.6547, -15.748) -> (115.8347, -15.748)
  line L99 (119.3125, -13.3521) -> (118.3689, -10.4819)
  line L100 (118.3689, -10.4819) -> (117.4303, -13.3521)
  line L101 (117.4303, -13.3521) -> (119.3125, -13.3521)
  line L102 (125.0528, -15.748) -> (121.5207, -15.748)
  line L103 (121.5207, -15.748) -> (121.5207, -9.652)
  line L104 (121.5207, -9.652) -> (122.3308, -9.652)
  line L105 (122.3308, -9.652) -> (122.3308, -15.0268)
  line L106 (122.3308, -15.0268) -> (125.0528, -15.0268)
  line L107 (125.0528, -15.0268) -> (125.0528, -15.748)
  line L108 (130.1361, -15.748) -> (129.0839, -15.748)
  line L109 (129.0839, -15.748) -> (126.8559, -12.9124)
  line L110 (126.8559, -12.9124) -> (126.5002, -13.3126)
  line L111 (126.5002, -13.3126) -> (126.5002, -15.748)
  line L112 (126.5002, -15.748) -> (125.6901, -15.748)
  line L113 (125.6901, -15.748) -> (125.6901, -9.652)
  line L114 (125.6901, -9.652) -> (126.5002, -9.652)
  line L115 (126.5002, -9.652) -> (126.5002, -12.453)
  line L116 (126.5002, -12.453) -> (128.9999, -9.652)
  line L117 (128.9999, -9.652) -> (129.9879, -9.652)
  line L118 (129.9879, -9.652) -> (127.4635, -12.374)
  line L119 (127.4635, -12.374) -> (130.1361, -15.748)
  dimension "d10" = 203.2
  dimension "d11" = 25.4
  dimension "d12" = 101.6
  dimension "d13" = 8.128
  dimension "d14" = 50.8
  dimension "d15" = 8.636
  constraints: 2 other
  measures "d10" distance of L2.start L1.end
  measures "d11" distance of L0.start L1.end
  measures "d12" distance of L4.start L4.end
  measures "d13" distance of L6.end L4.start
  measures "d14" distance between parallel lines of L1 L7
  measures "d15" distance between parallel lines of L2 L6
extrude "Extrusion3" cut sketch "Sketch3" against normal blind 2.54 contours L8 L9 L10 L11 L12 L13 | L14 L15 L16 L17 L18 L19 L20 L21 L22 L23 L24 L25 | S0 S1 L26 L27 L28 S2 S3 S4 L29 S5 | L36 L47 L43 | L43 L47 L48 L49 L50 L51 L52 L53 L54 | L36 L37 L38 L39 L40 L41 L42 S14 S15 S16 L43 L47 | L58 L59 L60 L61 L62 L63 L64 S21 S22 S23 L65 | L69 L70 L71 L72 L73 L74 L75 L76 L77 | L78 L79 L80 L81 L82 L83 L84 L85 L86 L87 L88 L89 L90 | L91 L92 L93 L94 L95 L96 L97 L98 | L102 L103 L104 L105 L106 L107 | L108 L109 L110 L111 L112 L113 L114 L115 L116 L117 L118 L119
sketch "Sketch4" plane through (203.2, 0, 50.8) normal (1, 0, 0) x (0, 0, -1)
  line L0 (0, 0) -> (50.8, 0) projected
  line L1 (0, 0) -> (0, -25.4) projected
  line L2 (50.8, -25.4) -> (0, -25.4) projected
  line L3 (50.8, 0) -> (50.8, -25.4) projected
  line L4 (12.7, -8.636) -> (38.1, -8.636) construction
  line L5 (38.1, -8.636) -> (38.1, -16.764) construction
  line L6 (38.1, -16.764) -> (12.7, -16.764) construction
  line L7 (12.7, -16.764) -> (12.7, -8.636) construction
  spline S0 degree 2 poles (15.0877, -15.8616) (14.4405, -15.8616) (13.3686, -15.4664) (12.9832, -15.0663) knots 0 0 0 1 2 2 2
  spline S1 degree 2 poles (12.9832, -15.0663) (12.5979, -14.6612) (12.1879, -13.4657) (12.1879, -12.6901) knots 0 0 0 1 2 2 2
  spline S2 degree 2 poles (12.1879, -12.6901) (12.1879, -11.9541) (12.6028, -10.7882) (12.9882, -10.3732) knots 0 0 0 1 2 2 2
  spline S3 degree 2 poles (12.9882, -10.3732) (13.3587, -9.9731) (14.4455, -9.5384) (15.0926, -9.5384) knots 0 0 0 1 2 2 2
  spline S4 degree 2 poles (15.0926, -9.5384) (15.4038, -9.5384) (15.967, -9.6273) (16.2239, -9.7063) knots 0 0 0 1 2 2 2
  spline S5 degree 2 poles (16.2239, -9.7063) (16.4314, -9.7656) (16.9353, -9.983) (17.0884, -10.062) knots 0 0 0 1 2 2 2
  line L8 (17.0884, -10.062) -> (17.0884, -11.0401)
  line L9 (17.0884, -11.0401) -> (17.0192, -11.0401)
  spline S6 degree 2 poles (17.0192, -11.0401) (16.8661, -10.9068) (16.545, -10.6647) (16.2486, -10.5264) knots 0 0 0 1 2 2 2
  spline S7 degree 2 poles (16.2486, -10.5264) (16.0016, -10.4029) (15.3643, -10.2399) (14.9988, -10.2399) knots 0 0 0 1 2 2 2
  spline S8 degree 2 poles (14.9988, -10.2399) (14.1194, -10.2399) (13.0326, -11.5638) (13.0326, -12.6654) knots 0 0 0 1 2 2 2
  spline S9 degree 2 poles (13.0326, -12.6654) (13.0326, -13.278) (13.3192, -14.1968) (13.5909, -14.513) knots 0 0 0 1 2 2 2
  spline S10 degree 2 poles (13.5909, -14.513) (13.8527, -14.8292) (14.5937, -15.1601) (15.058, -15.1601) knots 0 0 0 1 2 2 2
  spline S11 degree 2 poles (15.058, -15.1601) (15.3989, -15.1601) (16.0806, -15.0613) (16.3128, -14.9625) knots 0 0 0 1 2 2 2
  line L10 (16.3128, -14.9625) -> (16.3128, -13.3867)
  line L11 (16.3128, -13.3867) -> (14.9, -13.3867)
  line L12 (14.9, -13.3867) -> (14.9, -12.6753)
  line L13 (14.9, -12.6753) -> (17.1131, -12.6753)
  line L14 (17.1131, -12.6753) -> (17.1131, -15.338)
  spline S12 degree 2 poles (17.1131, -15.338) (16.96, -15.4071) (16.4363, -15.6196) (16.214, -15.6838) knots 0 0 0 1 2 2 2
  spline S13 degree 2 poles (16.214, -15.6838) (15.9127, -15.7727) (15.4285, -15.8616) (15.0877, -15.8616) knots 0 0 0 1 2 2 2
  line L15 (18.1307, -15.7431) -> (18.1307, -9.6471)
  line L16 (18.1307, -9.6471) -> (21.9444, -9.6471)
  line L17 (21.9444, -9.6471) -> (21.9444, -10.3683)
  line L18 (21.9444, -10.3683) -> (18.9409, -10.3683)
  line L19 (18.9409, -10.3683) -> (18.9409, -12.038)
  line L20 (18.9409, -12.038) -> (21.7419, -12.038)
  line L21 (21.7419, -12.038) -> (21.7419, -12.7593)
  line L22 (21.7419, -12.7593) -> (18.9409, -12.7593)
  line L23 (18.9409, -12.7593) -> (18.9409, -15.0218)
  line L24 (18.9409, -15.0218) -> (21.9444, -15.0218)
  line L25 (21.9444, -15.0218) -> (21.9444, -15.7431)
  line L26 (21.9444, -15.7431) -> (18.1307, -15.7431)
  line L27 (24.9579, -15.7431) -> (22.5965, -15.7431)
  line L28 (22.5965, -15.7431) -> (22.5965, -15.1206)
  line L29 (22.5965, -15.1206) -> (23.3721, -15.1206)
  line L30 (23.3721, -15.1206) -> (23.3721, -10.2695)
  line L31 (23.3721, -10.2695) -> (22.5965, -10.2695)
  line L32 (22.5965, -10.2695) -> (22.5965, -9.6471)
  line L33 (22.5965, -9.6471) -> (24.9579, -9.6471)
  line L34 (24.9579, -9.6471) -> (24.9579, -10.2695)
  line L35 (24.9579, -10.2695) -> (24.1823, -10.2695)
  line L36 (24.1823, -10.2695) -> (24.1823, -15.1206)
  line L37 (24.1823, -15.1206) -> (24.9579, -15.1206)
  line L38 (24.9579, -15.1206) -> (24.9579, -15.7431)
  spline S14 degree 2 poles (27.6601, -15.8517) (26.9981, -15.8517) (26.0694, -15.5751) (25.6594, -15.3775) knots 0 0 0 1 2 2 2
  line L39 (25.6594, -15.3775) -> (25.6594, -14.3599)
  line L40 (25.6594, -14.3599) -> (25.7186, -14.3599)
  spline S15 degree 2 poles (25.7186, -14.3599) (26.1188, -14.7353) (27.1315, -15.1503) (27.6008, -15.1503) knots 0 0 0 1 2 2 2
  spline S16 degree 2 poles (27.6008, -15.1503) (28.2726, -15.1503) (28.9593, -14.592) (28.9593, -14.1326) knots 0 0 0 1 2 2 2
  spline S17 degree 2 poles (28.9593, -14.1326) (28.9593, -13.767) (28.5987, -13.3126) (28.2084, -13.1989) knots 0 0 0 1 2 2 2
  spline S18 degree 2 poles (28.2084, -13.1989) (27.9268, -13.1199) (27.4575, -13.0112) (27.1068, -12.9223) knots 0 0 0 1 2 2 2
  spline S19 degree 2 poles (27.1068, -12.9223) (26.7906, -12.8383) (26.2917, -12.5864) (26.099, -12.3838) knots 0 0 0 1 2 2 2
  spline S20 degree 2 poles (26.099, -12.3838) (25.9113, -12.1813) (25.7038, -11.6379) (25.7038, -11.2822) knots 0 0 0 1 2 2 2
  spline S21 degree 2 poles (25.7038, -11.2822) (25.7038, -10.5412) (26.8598, -9.5384) (27.7539, -9.5384) knots 0 0 0 1 2 2 2
  spline S22 degree 2 poles (27.7539, -9.5384) (28.2677, -9.5384) (29.1767, -9.7409) (29.5669, -9.9336) knots 0 0 0 1 2 2 2
  line L41 (29.5669, -9.9336) -> (29.5669, -10.9018)
  line L42 (29.5669, -10.9018) -> (29.5076, -10.9018)
  spline S23 degree 2 poles (29.5076, -10.9018) (29.2162, -10.6351) (28.3072, -10.2399) (27.8083, -10.2399) knots 0 0 0 1 2 2 2
  spline S24 degree 2 poles (27.8083, -10.2399) (27.2451, -10.2399) (26.5486, -10.7684) (26.5486, -11.1982) knots 0 0 0 1 2 2 2
  spline S25 degree 2 poles (26.5486, -11.1982) (26.5486, -11.5836) (26.9586, -12.043) (27.3439, -12.1467) knots 0 0 0 1 2 2 2
  spline S26 degree 2 poles (27.3439, -12.1467) (27.6008, -12.2159) (28.3467, -12.3937) (28.5937, -12.4678) knots 0 0 0 1 2 2 2
  spline S27 degree 2 poles (28.5937, -12.4678) (29.2211, -12.6605) (29.804, -13.4361) (29.804, -14.0042) knots 0 0 0 1 2 2 2
  spline S28 degree 2 poles (29.804, -14.0042) (29.804, -14.3648) (29.5126, -15.0564) (29.2508, -15.2985) knots 0 0 0 1 2 2 2
  spline S29 degree 2 poles (29.2508, -15.2985) (28.9593, -15.5652) (28.2183, -15.8517) (27.6601, -15.8517) knots 0 0 0 1 2 2 2
  line L43 (30.629, -15.7431) -> (30.629, -9.6471)
  line L44 (30.629, -9.6471) -> (34.4427, -9.6471)
  line L45 (34.4427, -9.6471) -> (34.4427, -10.3683)
  line L46 (34.4427, -10.3683) -> (31.4392, -10.3683)
  line L47 (31.4392, -10.3683) -> (31.4392, -12.038)
  line L48 (31.4392, -12.038) -> (34.2402, -12.038)
  line L49 (34.2402, -12.038) -> (34.2402, -12.7593)
  line L50 (34.2402, -12.7593) -> (31.4392, -12.7593)
  line L51 (31.4392, -12.7593) -> (31.4392, -15.0218)
  line L52 (31.4392, -15.0218) -> (34.4427, -15.0218)
  line L53 (34.4427, -15.0218) -> (34.4427, -15.7431)
  line L54 (34.4427, -15.7431) -> (30.629, -15.7431)
  line L55 (38.8641, -15.7431) -> (35.3319, -15.7431)
  line L56 (35.3319, -15.7431) -> (35.3319, -9.6471)
  line L57 (35.3319, -9.6471) -> (36.1421, -9.6471)
  line L58 (36.1421, -9.6471) -> (36.1421, -15.0218)
  line L59 (36.1421, -15.0218) -> (38.8641, -15.0218)
  line L60 (38.8641, -15.0218) -> (38.8641, -15.7431)
  dimension "d18" = 50.8
  dimension "d19" = 25.4
  dimension "d20" = 25.4
  dimension "d21" = 8.128
  dimension "d22" = 8.636
  dimension "d23" = 12.7
  constraints: 2 other
  measures "d18" distance of L0.start L0.end
  measures "d19" distance of L0.start L1.end
  measures "d20" distance of L4.start L4.end
  measures "d21" distance of L6.end L4.start
  measures "d22" distance between parallel lines of L0 L4
  measures "d23" distance between parallel lines of L1 L7
extrude "Extrusion4" cut sketch "Sketch4" against normal blind 2.54 contours S0 S1 S2 S3 S4 S5 L8 L9 S6 S7 S8 S9 S10 S11 L10 L11 L12 L13 L14 S12 S13 | L15 L16 L17 L18 L19 L20 L21 L22 L23 L24 L25 L26 | L27 L28 L29 L30 L31 L32 L33 L34 L35 L36 L37 L38 | S14 L39 L40 S15 S16 S17 S18 S19 S20 S21 S22 L41 L42 S23 S24 S25 S26 S27 S28 S29 | L43 L44 L45 L46 L47 L48 L49 L50 L51 L52 L53 L54 | L55 L56 L57 L58 L59 L60